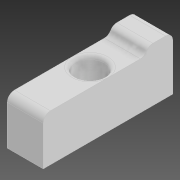
# Autodesk Inventor part: offset_vacuumbox
Saved by Autodesk Inventor 2020 (Build 240168000, 168)
## iProperties
Created: 2022-08-12
Part Number: offset_vacuumbox
Material: Generic
Document SubType Name: Modeling
Designer: Umair
Density: 1 g/cm^3
Appearance: Default
Author: Umair
Autodesk Inventor part; units mm, degrees
ref_plane "YZ Plane" through (0, 0, 0) normal (1, 0, 0) x (0, 1, 0)
ref_plane "XZ Plane" through (0, 0, 0) normal (0, 1, 0) x (-1, 0, 0)
ref_plane "XY Plane" through (0, 0, 0) normal (0, 0, 1) x (1, 0, 0)
sketch "Sketch1" plane through (0, 0, 0) normal (0, 1, 0) x (-1, 0, 0)
  line L0 (5, 18) -> (-5, 18)
  line L1 (-5, 18) -> (-5, -18)
  line L2 (-5, -18) -> (5, -18)
  line L3 (5, -18) -> (5, 18)
  line L4 (5, 18) -> (-5, -18) construction
  line L5 (-5, 18) -> (5, -18) construction
  line L6 (5, -18) -> (5, -11)
  line L7 (5, -11) -> (-5, -11)
  point P0 (0, 0)
  dimension "d0" = 10
  dimension "d1" = 36
  dimension "d2" = 7
  constraints: 16 end point, 2 midpoint, 2 parallel, 2 perpendicular, 2 point on line, 1 horizontal
  measures "d0" distance of L2.end L1.end
  measures "d1" distance of L1.end L0.end
  measures "d2" distance of L2.end L6.end
extrude "Extrusion1" add sketch "Sketch1" along normal blind 13 contours L3 L7 L1 L0
extrude "Extrusion2" add sketch "Sketch1" along normal blind 15 contours L3 L2 L1 L7
fillet "Fillet1" radius 2 4 edges at (0, 15, -11) (0, 13, -11) (0, 15, -18) (0, 13, 18)
sketch "Sketch2" plane through (0, 13, 0) normal (0, 1, 0) x (1, 0, 0)
  circle A0 centre (0, 0) radius 4
  circle A1 centre (0, 0) radius 2
  dimension "d8" = 8
  dimension "d9" = 4
  constraints: 2 centre point, 2 coincident
  measures "d8" diameter of A0
  measures "d9" diameter of A1
extrude "Extrusion3" cut sketch "Sketch2" against normal blind 15 contours A1
extrude "Extrusion4" cut sketch "Sketch2" against normal blind 10
fillet "Fillet2" radius 1 2 edges at (-2, 3, 0) (-4, 13, 0)
body "Solid1"
